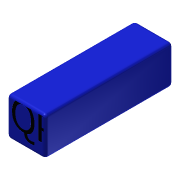
# Autodesk Inventor part: Container 2 2 5 colored color 1
Saved by Autodesk Inventor 2015 (Build 190159000, 159)
## iProperties
Created: 2015-03-07
Part Number: Container 2 2 5 colored color 1
Material: Generic
Document SubType Name: Modeling
Designer: Vukica
Density: 1 g/cm^3
Appearance: Blue - Wall Paint - Glossy
Author: Vukica
Autodesk Inventor part; units mm, degrees
ref_plane "YZ Plane" through (0, 0, 0) normal (1, 0, 0) x (0, 1, 0)
ref_plane "XZ Plane" through (0, 0, 0) normal (0, 1, 0) x (-1, 0, 0)
ref_plane "XY Plane" through (0, 0, 0) normal (0, 0, 1) x (1, 0, 0)
sketch "Sketch1" plane through (0, 0, 0) normal (0, 0, 1) x (1, 0, 0)
  line L0 (0, 0) -> (38.1, 0)
  line L1 (38.1, 0) -> (38.1, 38.1)
  line L2 (38.1, 38.1) -> (0, 38.1)
  line L3 (0, 38.1) -> (0, 0)
  dimension "d0" = 38.1
  dimension "d1" = 38.1
  constraints: 8 end point, 2 parallel, 1 horizontal, 1 perpendicular
  measures "d0" distance of L1.end L2.end
  measures "d1" distance of L2.end L0.start
extrude "Extrusion1" add sketch "Sketch1" along normal blind 127
sketch "Sketch2" plane through (0, 0, 127) normal (0, 0, 1) x (1, 0, 0)
  line L0 (-0.1987, 30.6387) -> (46.1964, 30.6387) construction
  line L1 (46.1964, 30.6387) -> (46.1964, -1.9861) construction
  line L2 (46.1964, -1.9861) -> (-0.1987, -1.9861) construction
  line L3 (-0.1987, -1.9861) -> (-0.1987, 30.6387) construction
  spline S0 degree 2 poles (18.7381, 4.9176) (17.9971, 4.7364) (16.3833, 4.5388) (15.5764, 4.5388) knots 0 0 0 1 2 2 2
  spline S1 degree 2 poles (15.5764, 4.5388) (13.2876, 4.5388) (10.4388, 7.0912) (10.3071, 9.4624) knots 0 0 0 1 2 2 2
  spline S2 degree 2 poles (10.3071, 9.4624) (10.1259, 9.4624) (9.8131, 9.4624) (9.6813, 9.4624) knots 0 0 0 1 2 2 2
  spline S3 degree 2 poles (9.6813, 9.4624) (7.623, 9.4624) (4.3132, 10.8621) (3.1276, 12.2288) knots 0 0 0 1 2 2 2
  spline S4 degree 2 poles (3.1276, 12.2288) (1.9584, 13.5791) (0.7069, 17.5311) (0.7069, 20.0341) knots 0 0 0 1 2 2 2
  spline S5 degree 2 poles (0.7069, 20.0341) (0.7069, 22.6029) (1.9749, 26.4891) (3.144, 27.8723) knots 0 0 0 1 2 2 2
  spline S6 degree 2 poles (3.144, 27.8723) (4.3296, 29.239) (7.6395, 30.6387) (9.6813, 30.6387) knots 0 0 0 1 2 2 2
  spline S7 degree 2 poles (9.6813, 30.6387) (11.7561, 30.6387) (15.0824, 29.1896) (16.2351, 27.8723) knots 0 0 0 1 2 2 2
  spline S8 degree 2 poles (16.2351, 27.8723) (17.3878, 26.5385) (18.6722, 22.57) (18.6722, 20.0341) knots 0 0 0 1 2 2 2
  spline S9 degree 2 poles (18.6722, 20.0341) (18.6722, 16.0821) (15.5929, 10.9444) (12.9088, 10.0387) knots 0 0 0 1 2 2 2
  spline S10 degree 2 poles (12.9088, 10.0387) (12.9747, 9.2813) (13.3699, 8.0627) (13.6828, 7.7169) knots 0 0 0 1 2 2 2
  spline S11 degree 2 poles (13.6828, 7.7169) (14.0615, 7.2888) (15.0989, 6.8936) (16.021, 6.8936) knots 0 0 0 1 2 2 2
  spline S12 degree 2 poles (16.021, 6.8936) (16.5644, 6.8936) (18.0465, 7.2394) (18.3758, 7.3711) knots 0 0 0 1 2 2 2
  line L4 (18.3758, 7.3711) -> (18.7381, 7.3711)
  line L5 (18.7381, 7.3711) -> (18.7381, 4.9176)
  spline S13 degree 2 poles (15.8564, 20.0341) (15.8564, 22.0595) (14.9836, 25.1717) (14.1932, 26.1927) knots 0 0 0 1 2 2 2
  spline S14 degree 2 poles (14.1932, 26.1927) (13.3864, 27.2465) (11.1139, 28.3004) (9.6978, 28.3004) knots 0 0 0 1 2 2 2
  spline S15 degree 2 poles (9.6978, 28.3004) (8.2323, 28.3004) (6.0257, 27.2795) (5.1859, 26.1927) knots 0 0 0 1 2 2 2
  spline S16 degree 2 poles (5.1859, 26.1927) (4.379, 25.1552) (3.5228, 22.0101) (3.5228, 20.0341) knots 0 0 0 1 2 2 2
  spline S17 degree 2 poles (3.5228, 20.0341) (3.5228, 16.0327) (6.882, 11.7678) (9.6978, 11.7678) knots 0 0 0 1 2 2 2
  spline S18 degree 2 poles (9.6978, 11.7678) (12.5136, 11.7678) (15.8564, 16.0327) (15.8564, 20.0341) knots 0 0 0 1 2 2 2
  line L6 (37.362, 9.8905) -> (33.8546, 9.8905)
  line L7 (33.8546, 9.8905) -> (27.4325, 17.9757)
  line L8 (27.4325, 17.9757) -> (24.3368, 17.9757)
  line L9 (24.3368, 17.9757) -> (24.3368, 9.8905)
  line L10 (24.3368, 9.8905) -> (21.6362, 9.8905)
  line L11 (21.6362, 9.8905) -> (21.6362, 30.2105)
  line L12 (21.6362, 30.2105) -> (26.8726, 30.2105)
  spline S19 degree 2 poles (26.8726, 30.2105) (28.6181, 30.2105) (30.9729, 29.8318) (32.0432, 29.1402) knots 0 0 0 1 2 2 2
  spline S20 degree 2 poles (32.0432, 29.1402) (33.1136, 28.4486) (34.3486, 26.2915) (34.3486, 24.6942) knots 0 0 0 1 2 2 2
  spline S21 degree 2 poles (34.3486, 24.6942) (34.3486, 22.4712) (32.0761, 19.4577) (30.1331, 18.7332) knots 0 0 0 1 2 2 2
  line L13 (30.1331, 18.7332) -> (37.362, 9.8905)
  spline S22 degree 2 poles (31.5327, 24.4801) (31.5327, 25.3693) (30.907, 26.7361) (30.2483, 27.1807) knots 0 0 0 1 2 2 2
  spline S23 degree 2 poles (30.2483, 27.1807) (29.672, 27.5594) (28.1406, 27.8723) (27.0208, 27.8723) knots 0 0 0 1 2 2 2
  line L14 (27.0208, 27.8723) -> (24.3368, 27.8723)
  line L15 (24.3368, 27.8723) -> (24.3368, 20.2317)
  line L16 (24.3368, 20.2317) -> (26.708, 20.2317)
  spline S24 degree 2 poles (26.708, 20.2317) (27.8771, 20.2317) (29.7379, 20.6434) (30.3801, 21.2856) knots 0 0 0 1 2 2 2
  spline S25 degree 2 poles (30.3801, 21.2856) (30.9729, 21.8454) (31.5327, 23.4262) (31.5327, 24.4801) knots 0 0 0 1 2 2 2
  point P0 (0, 0)
  constraints: 2 other
fillet "Fillet1" radius 3.175 4 edges at (38.1, 38.1, 63.5) (0, 38.1, 63.5) (0, 0, 63.5) (38.1, 0, 63.5)
fillet "Fillet2" radius 3.175 16 edges at (37.1701, 0.9299, 127) (38.1, 19.05, 127) (37.1701, 37.1701, 127) (19.05, 38.1, 127) (0.9299, 37.1701, 127) (0, 19.05, 127) (0.9299, 0.9299, 127) (19.05, 0, 127) (37.1701, 0.9299, 0) (38.1, 19.05, 0) (37.1701, 37.1701, 0) (19.05, 38.1, 0) (0.9299, 37.1701, 0) (0, 19.05, 0) (0.9299, 0.9299, 0) (19.05, 0, 0)
extrude "Extrusion3" cut sketch "Sketch2" against normal blind 0.254
body "Solid1"
